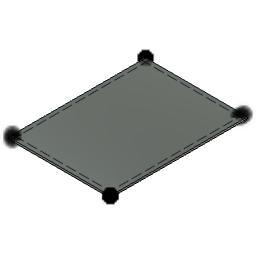
WordClock Rueckplatte (Autodesk Fusion 360 design; units mm, degrees)
Autodesk Fusion 360 part; units mm, degrees
sketch "Skizze1" plane through (0, 0, 0) normal (0, 0, 1) x (1, 0, 0)
  line L0 (-130, 175) -> (130, 175)
  line L1 (130, 175) -> (130, -175)
  line L2 (130, -175) -> (-130, -175)
  line L3 (-130, -175) -> (-130, 175)
  line L4 (-130, 175) -> (130, -175) construction
  line L5 (130, 175) -> (-130, -175) construction
  dimension "d1" = 260
  dimension "d2" = 350
  constraint horizontal L0
  constraint perpendicular L0 L1
  constraint parallel L0 L2
  constraint parallel L1 L3
  constraint coincident L4 origin
  constraint coincident L5 origin
  measures "d1" distance of L1.end L2.end
  measures "d2" distance of L0.end L1.end
extrude "Extrusion1" add sketch "Skizze1" along normal blind 5
sketch "Skizze2" plane through (0, 0, 5) normal (0, 0, 1) x (-1, 0, 0)
  line L0 (130, 175) -> (-130, 175)
  line L1 (-130, 175) -> (-130, -175)
  line L2 (-130, -175) -> (130, -175)
  line L3 (130, -175) -> (130, 175)
  line L4 (130, -175) -> (130, -165) construction
  line L5 (130, -175) -> (120, -175) construction
  line L6 (120, -175) -> (120, 175) construction
  line L7 (130, -165) -> (-130, -165) construction
  line L8 (-130, -165) -> (-120, -165) construction
  line L9 (-130, 175) -> (-120, 175) construction
  line L10 (-130, 175) -> (-130, 165) construction
  line L11 (-120, 175) -> (-120, -175) construction
  line L12 (-130, 165) -> (130, 165) construction
  dimension "d5" = 10
  dimension "d6" = 10
  dimension "d7" = 350
  dimension "d8" = 260
  dimension "d9" = 10
  dimension "d12" = 10
  dimension "d13" = 10
  dimension "d14" = 350
  dimension "d15" = 260
  constraint coincident L2.end L3.start
  constraint perpendicular L2 L4
  constraint perpendicular L3 L5
  constraint vertical L6
  constraint perpendicular L4 L7
  constraint perpendicular L1 L8
  constraint coincident L0.end L1.start
  constraint perpendicular L1 L9
  constraint perpendicular L9 L10
  constraint vertical L11
  constraint horizontal L12
  measures "d5" distance of L2.end L4.end
  measures "d6" distance of L2.end L5.end
  measures "d7" distance of L5.end L6.end
  measures "d8" distance of L4.end L7.end
  measures "d9" distance of L7.end L8.end
  measures "d12" distance of L0.end L9.end
  measures "d13" distance of L0.end L10.end
  measures "d14" distance of L9.end L11.end
  measures "d15" distance of L10.end L12.end
